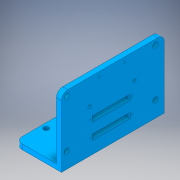
# Autodesk Inventor part: Realsense100
Saved by Autodesk Inventor 2019 (Build 230136000, 136)
## iProperties
Created: 2019-12-14
Part Number: Realsense100
Material: Generic
Document SubType Name: Modeling
Designer: james
Density: 1 g/cm^3
Appearance: Default(1)
Author: james
Autodesk Inventor part; units mm, degrees
ref_plane "YZ Plane" through (0, 0, 0) normal (1, 0, 0) x (0, 1, 0)
ref_plane "XZ Plane" through (0, 0, 0) normal (0, 1, 0) x (-1, 0, 0)
ref_plane "XY Plane" through (0, 0, 0) normal (0, 0, 1) x (1, 0, 0)
sketch "Sketch1" plane through (0, 0, 0) normal (1, 0, 0) x (0, 1, 0)
  line L0 (44.4049, 39.363) -> (-19.0951, 39.363)
  line L1 (-19.0951, 39.363) -> (-19.0951, -63.507)
  line L2 (-19.0951, -63.507) -> (44.4049, -63.507)
  line L3 (44.4049, -63.507) -> (44.4049, 39.363)
  point P0 (0, 0)
  dimension "d0" = 102.87
  dimension "d1" = 63.5
  constraints: 8 end point, 2 parallel, 1 horizontal, 1 perpendicular
  measures "d0" distance of L0.end L1.end
  measures "d1" distance of L0.start L0.end
extrude "Extrusion1" add sketch "Sketch1" along normal blind 5.08
sketch "Sketch2" plane through (5.08, 0, 0) normal (1, 0, 0) x (0, 0, -1)
  line L0 (63.507, 44.4049) -> (-39.363, 44.4049) projected
  line L1 (-39.363, 44.4049) -> (-39.363, -19.0951) projected
  point P0 (0, 0)
  point P1 (-34.283, 39.3249)
  point P2 (54.617, 39.3249)
  point P3 (54.617, -8.3001)
  point P4 (-34.283, -8.3001)
  dimension "d4" = 0
  dimension "d5" = 0
  dimension "d6" = 0
  dimension "d7" = 0
  dimension "d8" = 88.9
  dimension "d9" = 5.08
  dimension "d10" = 5.08
  dimension "d11" = 47.625
  measures "d4" horizontal distance of point (-34.283, -8.3) point (-34.283, 39.325)
  measures "d5" horizontal distance of point (54.617, -8.3) point (54.617, 39.325)
  measures "d6" vertical distance of point (-34.283, 39.325) point (54.617, 39.325)
  measures "d7" vertical distance of point (-34.283, -8.3) point (54.617, -8.3)
  measures "d8" distance of point (54.617, 39.325) point (-34.283, 39.325)
  measures "d9" distance from line of L0 point (-34.283, 39.325)
  measures "d10" distance from line of L1 point (-34.283, 39.325)
  measures "d11" distance of point (-34.283, -8.3) point (-34.283, 39.325)
hole "Hole1" at (5.08, 39.3249, 34.283) at (5.08, 39.3249, -54.617) at (5.08, -8.3001, -54.617) at (5.08, -8.3001, 34.283) direction (-1, 0, 0) diameter 5.1054 end through all clearance for "Flat Head Machine Screw (82)" size "#10" standard "Ansi Unified Screw Threads"
fillet "Fillet1" radius 6.35 2 edges at (2.54, 44.4049, 39.363) (2.54, 44.4049, -63.507)
sketch "Sketch7" plane through (0, -19.0951, 39.363) normal (0, 0, 1) x (1, 0, 0)
  line L0 (0, 0) -> (5.08, 0)
  line L1 (5.08, 0) -> (5.08, -5.08)
  line L2 (5.08, -5.08) -> (-40.64, -5.08)
  line L3 (-40.64, -5.08) -> (-40.64, 0)
  line L4 (-40.64, 0) -> (0, 0)
  line L5 (0, 0) -> (0, 0)
  line L6 (0, 0) -> (5.08, 0) projected
  line L7 (0, 57.15) -> (0, 0) projected
  point P0 (0, 19.0951)
  dimension "d51" = 5.08
  dimension "d52" = 5.08
  dimension "d53" = 90
  dimension "d54" = 5.08
  dimension "d55" = 45.72
  dimension "d56" = 0
  dimension "d57" = 0
  constraints: 12 end point, 3 perpendicular, 1 horizontal, 1 parallel
  measures "d51" distance of L0.start L0.end
  measures "d52" distance of L0.end L1.end
  measures "d53" angle of L2 L1
  measures "d54" distance of L2.end L3.end
  measures "d55" distance of L1.end L2.end
  measures "d56" distance between parallel lines of L0 L6
  measures "d57" distance between parallel lines of L7 L5
extrude "Extrusion4" add sketch "Sketch7" against normal blind 102.87
sketch "Sketch8" plane through (0, -19.0951, 39.363) normal (0, 1, 0) x (1, 0, 0)
  line L0 (0, 0) -> (0, 102.87) projected
  line L1 (-40.64, 0) -> (0, 0) projected
  line L2 (-40.64, 102.87) -> (0, 102.87) projected
  line L3 (-40.64, 0) -> (-40.64, 102.87) projected
  point P0 (0, 39.363)
  point P1 (-10.16, 25.4)
  point P2 (-35.56, 25.4)
  point P3 (-35.56, 76.2)
  point P4 (-10.16, 76.2)
  dimension "d67" = 0
  dimension "d69" = 0
  dimension "d71" = 0
  dimension "d72" = 0
  dimension "d143" = 5.08
  dimension "d144" = 26.67
  dimension "d145" = 50.8
  dimension "d146" = 25.4
  measures "d67" vertical distance of point (-35.56, 25.4) point (-10.16, 25.4)
  measures "d69" horizontal distance of point (-35.56, 25.4) point (-35.56, 76.2)
  measures "d71" vertical distance of point (-35.56, 76.2) point (-10.16, 76.2)
  measures "d72" horizontal distance of point (-10.16, 76.2) point (-10.16, 25.4)
  measures "d143" distance from line of L3 point (-35.56, 76.2)
  measures "d144" distance from line of L2 point (-35.56, 76.2)
  measures "d145" distance of point (-35.56, 25.4) point (-35.56, 76.2)
  measures "d146" distance of point (-10.16, 76.2) point (-35.56, 76.2)
hole "Hole3" at (-10.16, -19.0951, 13.963) at (-35.56, -19.0951, 13.963) at (-35.56, -19.0951, -36.837) at (-10.16, -19.0951, -36.837) direction (0, -1, 0) diameter 5.1054 end through all clearance for "Flat Head Machine Screw (82)" size "#10" standard "Ansi Unified Screw Threads"
fillet "Fillet2" radius 6.35 2 edges at (-40.64, -21.6351, -63.507) (-40.64, -21.6351, 39.363)
sketch "Sketch9" plane through (5.08, 0, 0) normal (1, 0, 0) x (0, 0, -1)
  line L0 (57.157, 44.4049) -> (-33.013, 44.4049) projected
  line L1 (-39.363, 38.0549) -> (-39.363, -24.1751) projected
  line L2 (63.507, 38.0549) -> (63.507, -24.1751) projected
  point P0 (0, 0)
  point P1 (-11.423, 19.0049)
  point P2 (33.577, 19.0049)
  dimension "d82" = 0
  dimension "d83" = 45
  dimension "d84" = 25.4
  dimension "d85" = 27.94
  dimension "d86" = 29.93
  measures "d82" vertical distance of point (-11.423, 19.005) point (33.577, 19.005)
  measures "d83" distance of point (33.577, 19.005) point (-11.423, 19.005)
  measures "d84" distance from line of L0 point (-11.423, 19.005)
  measures "d85" distance from line of L1 point (-11.423, 19.005)
  measures "d86" distance from line of L2 point (33.577, 19.005)
hole "Hole4" at (5.08, 19.0049, 11.423) at (5.08, 19.0049, -33.577) direction (-1, 0, 0) diameter 3.048 end through all
sketch "Sketch10" plane through (0, 0, 0) normal (-1, 0, 0) x (0, 0, 1)
  line L0 (-29.767, 41.8649) -> (8.333, 41.8649)
  line L1 (8.333, 41.8649) -> (8.333, 31.7049)
  line L2 (8.333, 31.7049) -> (-29.767, 31.7049)
  line L3 (-29.767, 31.7049) -> (-29.767, 41.8649)
  line L4 (-57.157, 44.4049) -> (33.013, 44.4049) projected
  circle A0 centre (-33.577, 19.0049) radius 1.524 projected
  circle A1 centre (11.423, 19.0049) radius 1.524 projected
  point P0 (0, 0)
  dimension "d94" = 10.16
  dimension "d95" = 38.1
  dimension "d96" = 2.54
  dimension "d97" = 3.81
  dimension "d98" = 3.09
  constraints: 8 end point, 2 parallel, 1 horizontal, 1 perpendicular
  measures "d94" distance of L2.end L0.start
  measures "d95" distance of L1.end L2.end
  measures "d96" distance between parallel lines of L4 L0
  measures "d97" distance from line of A0.centre L3
  measures "d98" distance from line of A1.centre L1
extrude "Extrusion5" add sketch "Sketch10" along normal blind 2.54 contours L0 L1 L2 L3
sketch "Sketch11" plane through (-2.54, 0, 0) normal (-1, 0, 0) x (0, 0, 1)
  line L0 (-29.767, 31.7049) -> (8.333, 31.7049) projected
  line L1 (-29.767, 41.8649) -> (-29.767, 31.7049) projected
  line L2 (8.333, 41.8649) -> (-29.767, 41.8649) projected
  line L3 (8.333, 31.7049) -> (8.333, 41.8649) projected
  point P0 (0, 0)
  point P1 (-23.417, 39.8329)
  point P2 (1.983, 39.8329)
  dimension "d101" = 0
  dimension "d102" = 25.4
  dimension "d103" = 6.35
  dimension "d104" = 8.128
  measures "d101" vertical distance of point (1.983, 39.833) point (-23.417, 39.833)
  measures "d102" distance of point (-23.417, 39.833) point (1.983, 39.833)
  measures "d103" distance from line of L1 point (-23.417, 39.833)
  measures "d104" distance from line of L0 point (-23.417, 39.833)
hole "Hole5" at (-2.54, 39.8329, -23.417) at (-2.54, 39.8329, 1.983) direction (1, 0, 0) diameter 1.778 end through all
sketch "Sketch12" plane through (5.08, 0, 0) normal (1, 0, 0) x (0, 0, -1)
  line L0 (-39.363, -24.1751) -> (63.507, -24.1751) projected
  line L1 (63.507, 38.0549) -> (63.507, -24.1751) projected
  point P0 (0, 0)
  point P1 (31.122, 6.8129)
  point P2 (-10.4756, 6.8129)
  point P3 (-10.4756, -8.9351)
  point P4 (31.122, -8.9351)
  dimension "d112" = 41.5976
  dimension "d113" = 0
  dimension "d114" = 0
  dimension "d115" = 15.748
  dimension "d116" = 0
  dimension "d117" = 0
  dimension "d118" = 15.24
  dimension "d119" = 32.385
  measures "d112" distance of point (-10.476, -8.935) point (31.122, -8.935)
  measures "d113" horizontal distance of point (-10.476, 6.813) point (-10.476, -8.935)
  measures "d114" horizontal distance of point (31.122, -8.935) point (31.122, 6.813)
  measures "d115" distance of point (31.122, -8.935) point (31.122, 6.813)
  measures "d116" vertical distance of point (-10.476, 6.813) point (31.122, 6.813)
  measures "d117" vertical distance of point (31.122, -8.935) point (-10.476, -8.935)
  measures "d118" distance from line of L0 point (31.122, -8.935)
  measures "d119" distance from line of L1 point (31.122, 6.813)
hole "Hole6" at (5.08, 6.8129, -31.122) at (5.08, 6.8129, 10.4756) at (5.08, -8.9351, 10.4756) at (5.08, -8.9351, -31.122) direction (-1, 0, 0) diameter 1 end through all
sketch "Sketch14" plane through (5.08, 0, 0) normal (1, 0, 0) x (0, 0, -1)
  line L0 (-8.6976, 9.3529) -> (29.344, 9.3529)
  line L1 (29.344, 9.3529) -> (29.344, 4.2729)
  line L2 (29.344, 4.2729) -> (-8.6976, 4.2729)
  line L3 (-8.6976, 4.2729) -> (-8.6976, 9.3529)
  line L4 (-8.6976, -6.3951) -> (29.344, -6.3951)
  line L5 (29.344, -6.3951) -> (29.344, -11.4751)
  line L6 (29.344, -11.4751) -> (-8.6976, -11.4751)
  line L7 (-8.6976, -11.4751) -> (-8.6976, -6.3951)
  circle A0 centre (31.122, -8.9351) radius 0.5 projected
  circle A1 centre (31.122, 6.8129) radius 0.5 projected
  circle A2 centre (-10.4756, 6.8129) radius 0.5 projected
  circle A3 centre (-10.4756, -8.9351) radius 0.5 projected
  point P0 (0, 0)
  dimension "d133" = 2.54
  dimension "d134" = 2.54
  dimension "d135" = 1.778
  dimension "d136" = 1.778
  dimension "d137" = 0
  dimension "d138" = 0
  dimension "d139" = 2.54
  dimension "d140" = 2.54
  constraints: 16 end point, 4 parallel, 2 horizontal, 2 perpendicular
  measures "d133" distance from line of A2.centre L2
  measures "d134" distance from line of L0 A2.centre
  measures "d135" distance from line of L3 A2.centre
  measures "d136" distance from line of L1 A1.centre
  measures "d137" distance between parallel lines of L7 L3
  measures "d138" distance between parallel lines of L5 L1
  measures "d139" distance from line of L4 A0.centre
  measures "d140" distance from line of L6 A0.centre
extrude "Extrusion7" cut sketch "Sketch14" against normal blind 20.725 contours L0 L1 L2 L3 | L4 L5 L6 L7
body "Solid1"
